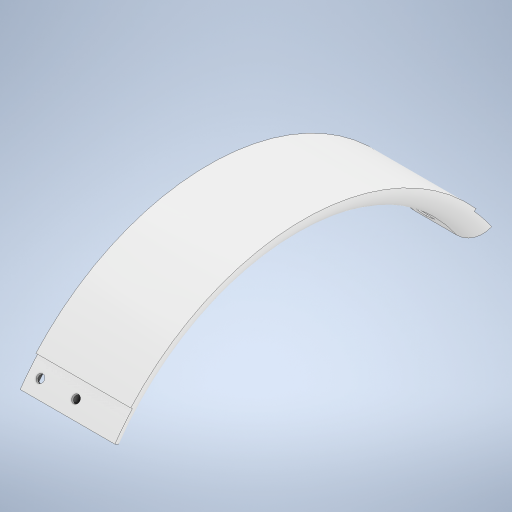
# Autodesk Inventor part: Ventilator_Flansch_Unten
Saved by Autodesk Inventor 2023 (Build 270158000, 158)
## iProperties
Created: 2022-12-27
Part Number: Ventilator_Flansch_Unten
Material: Generisch
Document SubType Name: Modeling
Designer: trist
Density: 1 g/cm^3
Appearance: Weiß
Author: trist
Autodesk Inventor part; units mm, degrees
ref_plane "XY Plane" through (0, 0, 0) normal (0, 0, 1) x (1, 0, 0)
sketch "Skizze6" plane through (0, 0, 0) normal (0, 0, 1) x (0, 1, 0)
  line L0 (0, 181.4954) -> (0, -165.4211)
  line L1 (196, 0) -> (196, -80)
  line L2 (179, -27) -> (179, -63)
  arc A0 (191, 0) -> (179, -27) centre (215.375, -27) ccw
  arc A1 (179, -63) -> (196, -80) centre (196, -63) ccw
  line L3 (191, 0) -> (196, 0)
  line L4 (258.45, 0) -> (-43.075, 0) projected
  point P0 (0, 0)
  dimension "d29" = 80
  dimension "d30" = 392
  dimension "d31" = 358
  dimension "d32" = 5
  dimension "d35" = 27
  constraints: 8 end point, 4 point on circle, 3 point on line, 3 vertical, 2 centre point, 2 tangent, 1 horizontal
  measures "d29" distance of L1.start L1.end
  measures "d30" diameter of L1 L0
  measures "d31" diameter of L2 L0
  measures "d32" distance of L3.start L1.start
  measures "d35" vertical distance of L2.start L3.start
revolve "Umdrehung1" add sketch "Skizze6" angle 110 mid plane about axis through (-181.4954, 0, 0) along (1, 0, 0)
ref_plane "Arbeitsebene1" through (10, 0, 0) normal (1, 0, 0) x (0, 1, 0)
sketch "Skizze7" plane through (10, 0, 0) normal (1, 0, 0) x (0, 1, 0)
  line L0 (0, 0) -> (200, 251.4345)
  line L1 (-40, 0) -> (240, 0) projected
  arc A0 (112.421, -160.5538) -> (112.421, 160.5538) centre (0, 0) ccw projected
  line L2 (122.0129, 153.3912) -> (119.5085, 155.3832)
  line L3 (119.5085, 155.3832) -> (117.0185, 152.2528)
  line L4 (117.0185, 152.2528) -> (116.3924, 152.7508)
  line L5 (116.3924, 152.7508) -> (108.2719, 142.5419)
  arc A1 (102.6702, -146.6282) -> (102.6702, 146.6282) centre (0, 0) ccw projected
  line L6 (108.2719, 142.5419) -> (111.4023, 140.0519)
  arc A2 (112.421, -160.5538) -> (112.421, 160.5538) centre (0, 0) ccw projected
  point P0 (111.4301, 140.0869)
  point P1 (119.4923, 155.3628)
  point P2 (122.0129, 153.3912)
  dimension "d37" = 51.5
  dimension "d38" = 200
  dimension "d39" = 6.4
  dimension "d40" = 8
  dimension "d41" = 4
  constraints: 12 end point, 4 perpendicular, 2 point on circle, 2 point on line, 1 other
  measures "d37" angle to the sketch x axis of L0
  measures "d38" horizontal distance of L0.start L0.end
  measures "d39" diameter of L3 L0
  measures "d40" diameter of L5 L0
  measures "d41" distance of L2.end L3.end
revolve "Umdrehung2" cut sketch "Skizze7" angle 360 about axis through (10, 0, 0) along (0, 0.6225146, 0.7826082) contours A1 L5 L4 L3 A0 L0 | A0 L3 L2
sketch "Skizze8" plane through (10, 119.5228, 150.2608) normal (0, -0.6225146, -0.7826082) x (1, 0, 0)
  line L0 (-5.2, -3.0022) -> (-5.2, 3.0022)
  line L1 (-5.2, 3.0022) -> (0, 6.0044)
  line L2 (0, 6.0044) -> (5.2, 3.0022)
  line L3 (5.2, 3.0022) -> (5.2, -3.0022)
  line L4 (5.2, -3.0022) -> (0, -6.0044)
  line L5 (0, -6.0044) -> (-5.2, -3.0022)
  line L6 (0, 74.1835) -> (0, -307.9253) projected
  circle A0 centre (0, 0) radius 3.2 projected
  line L7 (5.2, 3.0022) -> (10.4, 0)
  line L8 (10.4, 0) -> (5.2, -3.0022)
  point P0 (-10, 0)
  dimension "d43" = 10.4
  constraints: 16 end point, 2 point on line, 1 coincident, 1 collinear, 1 vertical, 13 other
  measures "d43" distance between parallel lines of L0 L3
extrude "Extrusion6" cut sketch "Skizze8" along normal blind 100 contours L0 L1 L6 A0 L5 | L6 A0 L2 L3 L4 | L3 L7 L8
pattern_linear "Rechteckige Anordnung1" count 2 spacing 30 along (1, 0, 0) of "Umdrehung2", "Extrusion6"
mirror "Spiegeln2" about plane through (0, 0, 0) normal (0, 0, 1) of "Umdrehung2", "Extrusion6", "Rechteckige Anordnung1"
sketch "Skizze11" plane through (0, 0, 0) normal (1, 0, 0) x (0, 1, 0)
  arc A0 (112.421, -160.5538) -> (112.421, 160.5538) centre (0, 0) ccw projected
  line L0 (112.421, 160.5538) -> (109.5531, 156.458) projected
  line L1 (112.421, -160.5538) -> (109.5531, -156.458) projected
  line L2 (0, 0) -> (131.1496, 145.6564)
  arc A1 (129.8113, 144.1701) -> (111.2738, 158.9155) centre (0, 0) ccw
  line L3 (-39, 0) -> (234, 0) projected
  point P0 (0, 0)
  dimension "d62" = 48
  dimension "d63" = 194
  constraints: 3 point on circle, 2 end point, 2 point on line, 1 centre point, 1 coincident
  measures "d62" angle of L3 L2
  measures "d63" radius of A1
extrude "Extrusion8" cut sketch "Skizze11" along normal through all contours L2 A1 L0 A0
mirror "Spiegeln3" about plane through (0, 0, 0) normal (0, 0, 1) of "Extrusion8"
ref_plane "Arbeitsebene4" through (40, 196, 0) normal (0, 1, 0) x (-1, 0, 0)
